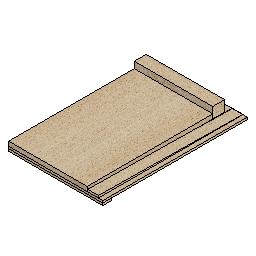
model (Autodesk Fusion 360 design; units mm, degrees)
Autodesk Fusion 360 part; units mm, degrees
sketch "Sketch1" plane through (0, 0, 0) normal (0, 0, 1) x (1, 0, 0)
  line L0 (0, 0) -> (320, 0)
  line L1 (320, 0) -> (320, 512.5)
  line L2 (320, 512.5) -> (0, 512.5)
  line L3 (0, 512.5) -> (0, 0)
  line L4 (0, 512.5) -> (0, 589.5)
  line L5 (0, 589.5) -> (384, 589.5)
  line L6 (384, 589.5) -> (384, 0)
  line L7 (384, 0) -> (320, 0)
  line L8 (0, 561) -> (320, 561)
  line L9 (320, 561) -> (320, 512.5)
  line L10 (322.5, 589.5) -> (322.5, 0)
  line L11 (366, 0) -> (366, 589.5)
  line L12 (0, 37) -> (384, 37)
  dimension "d1" = 512.5
  dimension "d2" = 320
  dimension "d3" = 77
  dimension "d4" = 64
  dimension "d5" = 48.5
  dimension "d6" = 43.5
  dimension "d7" = 2.5
  dimension "d18" = 37
  constraint horizontal L0
  constraint vertical L1
  constraint horizontal L2
  constraint vertical L3
  constraint coincident L0.start L3.end
  constraint horizontal L7
  constraint vertical L6
  constraint horizontal L5
  constraint vertical L4
  constraint coincident L4 L8.start
  constraint vertical L9
  constraint horizontal L8
  constraint coincident L5 L10.start
  constraint coincident L7 L10.end
  constraint coincident L7 L11.start
  constraint coincident L5 L11.end
  constraint vertical L10
  constraint vertical L11
  constraint coincident L3 L12.start
  constraint coincident L6 L12.end
  constraint horizontal L12
  measures "d1" distance of L0.start L2.end
  measures "d2" distance of L0.start L0.end
  measures "d3" distance of L2.end L4.end
  measures "d4" distance of L1 L6
  measures "d5" distance of L2 L8
  measures "d6" distance of L10 L11
  measures "d7" distance of L1 L10
  measures "d18" distance of L0 L12
extrude "Extrude1" add sketch "Sketch1" against normal blind 9 makes body 1
extrude "Extrude2" add sketch "Sketch1" along normal blind 18 separate body contours L0 L1 L3 L12 | L1 L2 L3 L12 makes body 2
extrude "Extrude3" add sketch "Sketch1" along normal blind 44 separate body contours L2 L4 L8 L9 makes body 3
extrude "Extrude4" add sketch "Sketch1" along normal blind 9 separate body contours L7 L10 L11 L12 | L5 L10 L11 L12 makes body 4
draft "Draft1" angle -0.8 neutral plane through (366, 0, 0) pull (0, -1, 0) 1 faces at (337, 405.3333, 9) on bodies 4
extrude "Extrude5" add sketch "Sketch1" against normal blind 9 from surface at -9 separate body contours L0 L1 L3 L12 | L1 L7 L10 L12 | L7 L10 L11 L12 | L6 L7 L11 L12 makes body 5
